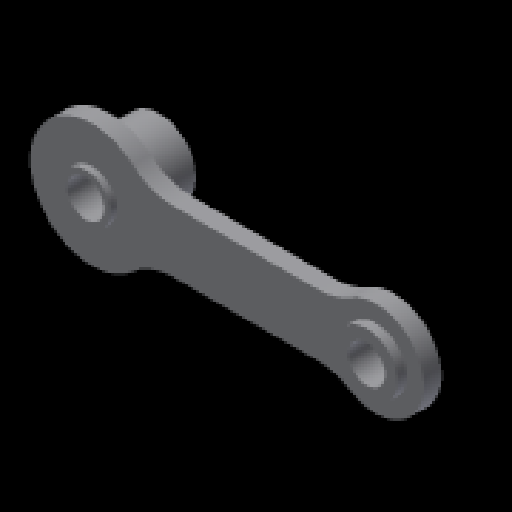
# Autodesk Inventor part: LegChainTensionerArm
Saved by Autodesk Inventor 2025.2 (Build 292293000, 293)
## iProperties
Created: 2026-01-19
Part Number: LegChainTensionerArm
Material: Generic
Document SubType Name: Sheet Metal
Designer: valer
Density: 1 g/cm^3
Sheet Metal Rule: Default_mm
Appearance: Default
Author: valer
Autodesk Inventor part; units mm, degrees
ref_plane "YZ Plane" through (0, 0, 0) normal (1, 0, 0) x (0, 1, 0)
ref_plane "XZ Plane" through (0, 0, 0) normal (0, 1, 0) x (-1, 0, 0)
ref_plane "XY Plane" through (0, 0, 0) normal (0, 0, 1) x (1, 0, 0)
sketch "Base" plane through (0, 0, 0) normal (0, 0, 1) x (1, 0, 0)
  circle A0 centre (0, 0) radius 10
  line L0 (0, 0) -> (46, 0) construction
  circle A1 centre (46, 0) radius 7.75
  line L1 (8.6603, 5) -> (40.0786, 5)
  line L2 (40.0786, 5) -> (40.0786, -5)
  line L3 (40.0786, -5) -> (8.6603, -5)
  line L4 (8.6603, -5) -> (8.6603, 5)
  circle A2 centre (46, 0) radius 3
  circle A3 centre (0, 0) radius 3
  point P0 (8.6603, 0)
  point P1 (8.6603, -5)
  dimension "d0" = 20
  dimension "d2" = 15.5
  dimension "d1" = 46
  dimension "d3" = 10
  dimension "d4" = 6
  dimension "d5" = 6
  measures "d1" distance of L0.start L0.end
  measures "d3" distance of L3.end L1.start
  measures "d4" diameter of A2
  measures "d5" diameter of A3
extrude "Plate1" add sketch "Base" along normal blind 2.9
sketch "Shoulder" plane through (0, 0, 0) normal (0, 0, -1) x (-1, 0, 0)
  circle A0 centre (0, 0) radius 3 projected
  circle A1 centre (0, 0) radius 3 projected
  circle A2 centre (0, 0) radius 6
  circle A3 centre (0, 0) radius 4
  dimension "d7" = 12
  dimension "d8" = 2
  constraints: 2 centre point, 2 coincident
  measures "d7" diameter of A2
  measures "d8" radial gap between concentric circles of A2 A3
extrude "ShoulderFeature" add sketch "Shoulder" along normal blind 8 contours A2
sketch "Mount" plane through (0, 0, 2.9) normal (0, 0, 1) x (1, 0, 0)
  circle A0 centre (46, 0) radius 3 projected
  circle A1 centre (46, 0) radius 5
  point P0 (0, 0)
  dimension "d11" = 2
  constraints: 1 centre point, 1 coincident
  measures "d11" radial gap between concentric circles of A1 A0
extrude "MountFeature" add sketch "Mount" along normal blind 1.5
fillet "BaseFilletsFeature" radius 10 2 edges at (8.6603, 5, 1.45) (8.6603, -5, 1.45)
fillet "EndFilletsFeature" radius 10 2 edges at (40.0786, 5, 1.45) (40.0786, -5, 1.45)
sketch "Sketch6" plane through (0, 0, 2.9) normal (0, 0, 1) x (1, 0, 0)
  circle A0 centre (0, 0) radius 3 projected
  circle A1 centre (0, 0) radius 4
  dimension "d17" = 1
  constraints: 1 centre point, 1 coincident
  measures "d17" radial gap between concentric circles of A1 A0
extrude "Extrusion3" add sketch "Sketch6" along normal blind 1
equation "\"d6\" = Thickness"
equation "\"BendRadius\" = Thickness"
equation "\"BendReliefWidth\" = Thickness"
equation "\"BendReliefDepth\" = 0.5 * Thickness"
equation "\"CornerReliefSize\" = 4 * Thickness"
equation "\"MinimumRemnant\" = 2 * Thickness"
equation "\"TransitionRadius\" = BendRadius"
equation "\"JacobiRadiusSize\" = BendRadius"
equation "\"GapSize\" = Thickness"
equation "\"Thickness\" = 2.9"
body "Solid1"
